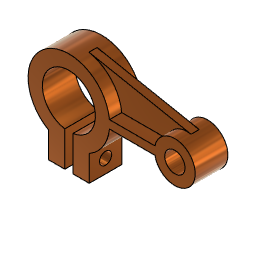
Exercise-8 v1 (Autodesk Fusion 360 design; units mm, degrees)
Autodesk Fusion 360 part; units mm, degrees
sketch "Sketch1" plane through (0, 0, 0) normal (0, 1, 0) x (1, 0, 0)
  circle A0 centre (130, 0) radius 12.5
  circle A1 centre (130, 0) radius 25
  line L0 (-5, 32.1131) -> (-5, 75.0003)
  line L1 (5, 75.0003) -> (5, 32.1131)
  line L2 (25, 43.3013) -> (25, 75.0003)
  line L3 (-25, 75.0003) -> (-25, 43.3013)
  line L4 (49.7494, -5) -> (105.5051, -5)
  line L5 (105.5051, 5) -> (49.7494, 5)
  line L6 (-127.7852, 0) -> (32.5, 0) construction
  line L7 (117.5, 0) -> (145, 0) construction
  line L8 (0, -32.5) -> (0, -85) construction
  line L9 (0, 28.4863) -> (0, 0) construction
  arc A2 (-4.3331, 32.2098) -> (4.3331, 32.2098) centre (0, 0) ccw
  arc A3 (-25, 43.3013) -> (25, 43.3013) centre (0, 0) ccw
  line L10 (25, 75.0003) -> (5, 75.0003)
  line L11 (-5, 75.0003) -> (-25, 75.0003)
  line L12 (9.6154, -49.0667) -> (134.8077, -24.5334)
  dimension "d1" = 65
  dimension "d3" = 25
  dimension "d4" = 50
  dimension "d6" = 50
  dimension "d7" = 31.699
  constraint coincident L9.end A2.centre
  constraint horizontal L6
  constraint coincident A0.centre L6
  constraint concentric A0 A1
  constraint parallel L0 L1
  constraint vertical L2
  constraint horizontal L10
  constraint vertical L3
  constraint horizontal L4
  constraint parallel L4 L5
  constraint coincident L6.end A2
  constraint coincident A1 L4.end
  constraint coincident A0 L7.start
  constraint coincident A1 L5.start
  constraint coincident L6 L9.end
  constraint coincident L8.start A2
  constraint coincident A2 L0.start
  constraint coincident A2 L1.end
  constraint collinear L10 L11
  constraint coincident A3 L12.start
  constraint tangent A3 L12
  constraint coincident A1 L12.end
  constraint tangent A1 L12
  measures "d1" diameter of A2
  measures "d3" diameter of A0
  measures "d4" diameter of A1
  measures "d6" distance of L3.end L2.start
  measures "d7" distance of L3.end L3.start
extrude "Extrude1" add sketch "Sketch1" along normal mid plane 40 contours A1 | A1 L4 L5 A3 | L0 L1 L2 L3 A2 A3 L10 L11
extrude "Extrude2" add sketch "Sketch1" along normal mid plane 10 contours A1 L4 A3 L12
hole "Hole1" at (25, 0, -58.3013) direction (-1, 0, 0) diameter 15 end through all
